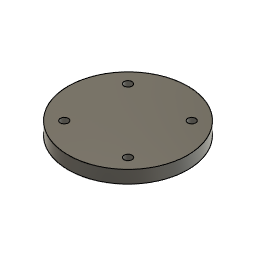
SupportBalise v3 (Autodesk Fusion 360 design; units mm, degrees)
Autodesk Fusion 360 part; units mm, degrees
sketch "Sketch1" plane through (0, 0, 0) normal (0, 1, 0) x (1, 0, 0)
  circle A0 centre (0, 0) radius 37.5
  line L0 (-20, 20) -> (20, 20) construction
  line L1 (20, 20) -> (20, -20) construction
  line L2 (20, -20) -> (-20, -20) construction
  line L3 (-20, -20) -> (-20, 20) construction
  line L4 (-20, 20) -> (20, -20) construction
  circle A1 centre (-20, 20) radius 2.5
  circle A2 centre (20, 20) radius 2.5
  circle A3 centre (-20, -20) radius 2.5
  circle A4 centre (20, -20) radius 2.5
  dimension "d1" = 75
  dimension "d2" = 40
  dimension "d3" = 40
  dimension "d4" = 5
  dimension "d5" = 5
  dimension "d6" = 5
  dimension "d7" = 5
  constraint coincident A0.centre origin
  constraint horizontal L0
  constraint vertical L1
  constraint horizontal L2
  constraint vertical L3
  constraint midpoint A0.centre L4
  constraint coincident L0.start L3.end
  constraint coincident L0.end L1.start
  constraint coincident L2.end L3.start
  constraint coincident L1.end L2.start
  measures "d1" diameter of A0
  measures "d2" distance of L0.start L0.end
  measures "d3" distance of L0.start L2.end
  measures "d4" diameter of A1
  measures "d5" diameter of A2
  measures "d6" diameter of A3
  measures "d7" diameter of A4
extrude "Extrude1" add sketch "Sketch1" along normal blind 15
extrude "Extrude2" cut 1 faces at (-6.0558, 0, -6.0999) along direction (0, 1, 0) blind 7
equation "d10 = -15 mm + 8 mm"
named bodies: "SupportBalise"
